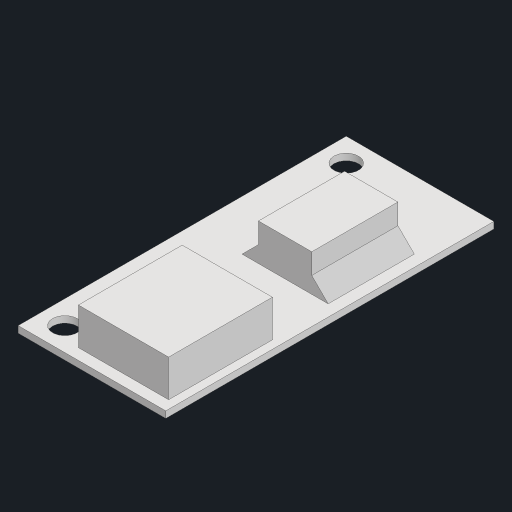
# Autodesk Inventor part: interface_board
Saved by Autodesk Inventor 2023 (Build 270158000, 158)
## iProperties
Created: 2024-04-13
Part Number: interface_board
Material: Generic
Document SubType Name: Modeling
Designer: szymo
Density: 1 g/cm^3
Appearance: Default
Author: szymo
Autodesk Inventor part; units mm, degrees
ref_plane "YZ Plane" through (0, 0, 0) normal (1, 0, 0) x (0, 1, 0)
ref_plane "XZ Plane" through (0, 0, 0) normal (0, 1, 0) x (-1, 0, 0)
ref_plane "XY Plane" through (0, 0, 0) normal (0, 0, 1) x (1, 0, 0)
sketch "Sketch1" plane through (0, 0, 0) normal (0, 1, 0) x (-1, 0, 0)
  line L0 (0, 0) -> (-18, 0)
  line L1 (-18, 0) -> (-18, -40)
  line L2 (-18, -40) -> (0, -40)
  line L3 (0, -40) -> (0, 0)
  line L4 (-1.35, 0) -> (-1.35, -40)
  line L5 (0, -1.35) -> (-18, -1.35)
  line L6 (0, -38.65) -> (-18, -38.65)
  circle A0 centre (-2.85, -2.85) radius 1.5
  circle A1 centre (-2.85, -37.15) radius 1.5
  line L7 (-8.1, -21.2) -> (-14.6, -21.2)
  line L8 (-14.6, -21.2) -> (-14.6, -31.7)
  line L9 (-14.6, -31.7) -> (-8.1, -31.7)
  line L10 (-8.1, -31.7) -> (-8.1, -21.2)
  line L11 (-6, -1) -> (-17, -1)
  line L12 (-17, -1) -> (-17, -14)
  line L13 (-17, -14) -> (-6, -14)
  line L14 (-6, -14) -> (-6, -1)
  point P0 (-6, -1.35)
  point P1 (-17, -1.35)
  dimension "d0" = 18
  dimension "d1" = 40
  dimension "d2" = 1.35
  dimension "d3" = 1.35
  dimension "d4" = 1.35
  dimension "d5" = 3
  dimension "d6" = 3
  dimension "d7" = 6.5
  dimension "d8" = 10.5
  dimension "d11" = 8.1
  dimension "d12" = 8.3
  dimension "d13" = 11
  dimension "d14" = 13
  dimension "d16" = 1
  dimension "d17" = 1
  constraints: 30 end point, 6 parallel, 6 perpendicular, 6 point on line, 4 tangent, 3 horizontal, 2 centre point
  measures "d0" distance of L2.end L1.end
  measures "d1" distance of L1.end L0.end
  measures "d2" distance between parallel lines of L4 L3
  measures "d3" distance between parallel lines of L0 L5
  measures "d4" distance between parallel lines of L6 L2
  measures "d5" diameter of A0
  measures "d6" diameter of A1
  measures "d7" distance of L9.end L8.end
  measures "d8" distance of L8.end L7.end
  measures "d11" distance between parallel lines of L3 L10
  measures "d12" distance between parallel lines of L2 L9
  measures "d13" distance of L12.end L13.end
  measures "d14" distance of L13.end L11.start
  measures "d16" distance between parallel lines of L0 L11
  measures "d17" distance between parallel lines of L12 L1
extrude "Extrusion1" add sketch "Sketch1" against normal blind 0.8 contours L3 L5 L4 L0 | L4 L5 L14 L11 L12 L1 L0 | L3 L6 L4 L5 | L4 A0 L5 | L3 L2 L4 L6 | L5 L12 L13 L14 A0 L4 A1 L6 L1 | L6 A1 L4 | L4 L2 L1 L6 | L12 L11 L14 L5 | L5 L14 L13 L12 | L10 L9 L8 L7
extrude "Extrusion2" add sketch "Sketch1" along normal blind 4.5 contours L5 L14 L13 L12
extrude "Extrusion3" add sketch "Sketch1" along normal blind 4.5 contours L10 L9 L8 L7
chamfer "Chamfer1" distance 2 angle 45 2 edges at (8.1, 0, -26.45) (14.6, 0, -26.45)
body "Solid1"
